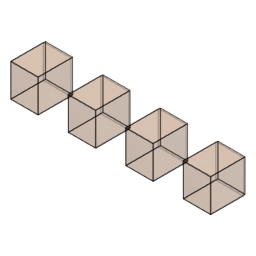
Finger Joint (Autodesk Fusion 360 design; units mm, degrees)
Autodesk Fusion 360 part; units mm, degrees
sketch "Contact Patch" plane through (0, 0, 0) normal (0, 0, 1) x (1, 0, 0)
  line L0 (75, 9) -> (-75, 9)
  line L1 (-75, 9) -> (-75, -9)
  line L2 (-75, -9) -> (75, -9)
  line L3 (75, -9) -> (75, 9)
  line L4 (75, 9) -> (-75, -9) construction
  line L5 (-75, 9) -> (75, -9) construction
  dimension "d5" = 18
  dimension "d6" = 150
  constraint horizontal L0
  constraint perpendicular L0 L1
  constraint parallel L0 L2
  constraint parallel L1 L3
  constraint coincident L4 origin
  constraint coincident L5 origin
  measures "d5" distance of L0.end L1.end
  measures "d6" distance of L1.end L2.end
ref_plane "WorkPlane1" through (0, 0, 18.1) normal (0, 0, 1) x (1, 0, 0)
sketch "Sketch2" plane through (0, 0, 18.1) normal (0, 0, 1) x (1, 0, 0)
  line L0 (-55, 8.9999) -> (-40, 8.9999)
  line L1 (-40, 8.9999) -> (-40, -8.9999)
  line L2 (-40, -8.9999) -> (-55, -8.9999)
  line L3 (-55, -8.9999) -> (-55, 8.9999)
  line L4 (-75, 9) -> (-75, -9)
  line L5 (75, 9) -> (-75, 9)
  line L6 (-75, -9) -> (75, -9)
  dimension "d45" = 20
  dimension "d46" = 15
  dimension "d47" = 0.0001
  dimension "d48" = 0.0001
  constraint horizontal L0
  constraint vertical L1
  constraint horizontal L2
  constraint vertical L3
  measures "d45" distance of L3 L4
  measures "d46" distance of L0.start L0.end
  measures "d47" distance of L0 L5
  measures "d48" distance of L2 L6
extrude "Extrude1" add sketch "Sketch2" against normal up to surface (18.1 mm away) contours L0 L1 L2 L3 L5 L6 makes body 1
move_face "OffsetFaces1" offset 1 1 faces at (-50, 3, 0) on bodies 1
ref_plane "WorkPlane2" through (0, -9, 0) normal (0, 1, 0) x (0, 0, 1)
sketch "Sketch3" plane through (0, 0, 0) normal (0, 1, 0) x (0, 0, 1)
  line L0 (-1, -40) -> (-1, -55)
  line L1 (-1, -55) -> (18.1, -55)
  line L2 (18.1, -55) -> (18.1, -40)
  line L3 (18.1, -40) -> (-1, -40)
  line L4 (0, -55) -> (0, -40)
  constraint coincident L1 L4.start
  constraint coincident L3 L4.end
  constraint perpendicular L3 L4
extrude "Extrude2" add sketch "Sketch3" along normal blind 8.9999 and the other way blind 8.9999 separate body contours L1 L2 L3 L4 makes body 2
move_face "OffsetFaces3" offset 0.001 1 faces at (-50, -3, 18.1) on bodies 2
move_face "OffsetFaces4" offset 0.2 4 faces at (-55, 3, 6.0337) (-45, 8.9999, 6.0337) (-40, 3, 12.0673) (-45, -8.9999, 6.0337) on bodies 2
copy_body "CutPasteBodies1" bodies 1 2 removing the originals makes body 3 makes body 4 in component "Joint"
pattern_linear "00000000-0000-0000-0000-000000000000" [suppressed]
component "Joint" placed x (1, 0, 0) y (0, 1, 0) z (0, 0, 1) at (0, 0, 0)
component "Joint" placed x (1, 0, 0) y (0, 1, 0) z (0, 0, 1) at (31.6667, 0, 0)
component "Joint" placed x (1, 0, 0) y (0, 1, 0) z (0, 0, 1) at (63.3333, 0, 0)
component "Joint" placed x (1, 0, 0) y (0, 1, 0) z (0, 0, 1) at (95, 0, 0)
equation "Length = 150 mm"
equation "Width = 18 mm"
equation "d5 = Width"
equation "d6 = Length"
equation "Nestled_T = 18 mm"
equation "Tenon_Height = Nestled_T + 0.1 mm" comment "Board Height plus clearance"
equation "d9 = Tenon_Height"
equation "SideOffset1 = 0.0001 mm"
equation "SideOffset2 = 0.0001 mm"
equation "UserOffset1 = 20 mm"
equation "Tenon_Length = 15 mm"
equation "UserOffset2 = 20 mm"
equation "Offset1 = UserOffset1"
equation "Offset2 = UserOffset2"
equation "Tenon_QTY = 4"
equation "Spacing_Length = Length - Offset1 - Offset2 - Tenon_Length"
equation "d30 = -Width / 2"
equation "Mortise_width1 = ( Width / 2 ) - SideOffset1"
equation "Mortise_width2 = ( Width / 2 ) - SideOffset2"
equation "d33 = Mortise_width1"
equation "d35 = Mortise_width2"
equation "Clearance = 0.2 mm"
equation "d40 = Clearance"
equation "d45 = Offset1"
equation "d46 = Tenon_Length"
equation "d47 = SideOffset1"
equation "d48 = SideOffset2"
equation "d49 = Tenon_QTY"
equation "d51 = Spacing_Length"
named bodies: "Tenon", "Mortise"
